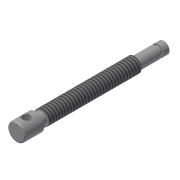
# Autodesk Inventor part: Vise_Screw
Saved by Autodesk Inventor 2022 (Build 260148000, 148)
## iProperties
Created: 2006-01-18
Part Number: Vise_Screw
Document SubType Name: Modeling
Designer: PMiller
Material: Steel, Mild
Density: 7.86 g/cm^3
Appearance: Steel
Author: PMiller
Autodesk Inventor part; units mm, degrees
ref_plane "YZ Plane" through (0, 0, 0) normal (1, 0, 0) x (0, 1, 0)
ref_plane "XZ Plane" through (0, 0, 0) normal (0, 1, 0) x (-1, 0, 0)
ref_plane "XY Plane" through (0, 0, 0) normal (0, 0, 1) x (1, 0, 0)
sketch "Sketch1" plane through (0, 0, 0) normal (0, 0, 1) x (1, 0, 0)
  line L0 (0, 158.75) -> (9.525, 158.75)
  line L1 (9.525, 158.75) -> (9.525, 138.1125)
  line L2 (9.525, 138.1125) -> (6.35, 138.1125)
  line L3 (6.35, 138.1125) -> (6.35, 131.7625)
  line L4 (6.35, 131.7625) -> (7.9375, 131.7625)
  line L5 (7.9375, 131.7625) -> (7.9375, 31.75)
  line L6 (7.9375, 31.75) -> (6.35, 31.75)
  line L7 (6.35, 31.75) -> (6.35, 9.6012)
  line L8 (6.35, 9.6012) -> (4.7625, 9.6012)
  line L9 (4.7625, 9.6012) -> (4.7625, 6.35)
  line L10 (4.7625, 6.35) -> (6.35, 6.35)
  line L11 (6.35, 6.35) -> (6.35, 0)
  line L12 (6.35, 0) -> (0, 0)
  line L13 (0, 0) -> (0, 158.75)
  dimension "d0" = 12.7
  dimension "d1" = 9.525
  dimension "d3" = 12.7
  dimension "d4" = 15.875
  dimension "d5" = 12.7
  dimension "d6" = 19.05
  dimension "d7" = 20.6375
  dimension "d8" = 6.35
  dimension "d9" = 100.0125
  dimension "d10" = 6.35
  dimension "d11" = 3.2512
  dimension "d12" = 158.75
  constraints: 28 end point, 12 parallel, 1 horizontal, 1 perpendicular
  measures "d0" diameter of L11 L13
  measures "d1" diameter of L9 L13
  measures "d3" diameter of L7 L13
  measures "d4" diameter of L5 L13
  measures "d5" diameter of L3 L13
  measures "d6" diameter of L1 L13
  measures "d7" distance of L0.end L1.end
  measures "d8" distance of L2.end L3.end
  measures "d9" distance of L4.end L5.end
  measures "d10" distance of L10.end L11.end
  measures "d11" distance of L8.end L9.end
  measures "d12" distance of L12.end L0.start
revolve "Revolution1" add sketch "Sketch1" angle 360 about axis through (0, 0, 0) along (0, 1, 0)
thread "Thread1" size "5/8-8 Acme" class "2G" standard "ACME" full length
sketch "Sketch2" plane through (0, 0, 0) normal (0, 0, 1) x (1, 0, 0)
  line L0 (-9.525, 158.75) -> (9.525, 158.75) projected
  circle A0 centre (0, 148.4313) radius 4.3656
  point P0 (0, 158.75)
  dimension "d16" = 8.7312
  dimension "d17" = 10.3187
  constraints: 1 centre point, 1 midpoint, 1 vertical alignment
  measures "d16" diameter of A0
  measures "d17" distance from line of L0 A0.centre
extrude "Extrusion1" cut sketch "Sketch2" along normal through all both and the other way through all
fillet "Fillet1" radius 1.5875 1 edges at (-9.525, 158.75, 0)
body "Solid1"
